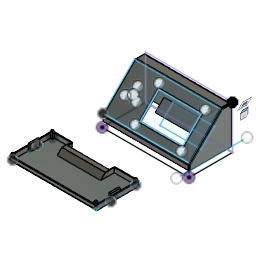
aether pad case split (Autodesk Fusion 360 design; units mm, degrees)
part number: 2026-05-05-17-50-19-673
Autodesk Fusion 360 part; units mm, degrees
sketch "Sketch1" plane through (0, 0, 0) normal (0, 0, 1) x (1, 0, 0)
  line L0 (0, 0) -> (180, 0)
  line L1 (180, 0) -> (180, 90)
  line L2 (180, 90) -> (0, 90)
  line L3 (0, 90) -> (0, 0)
  dimension "d1" = 180
  dimension "d2" = 90
  constraint horizontal L0
  constraint vertical L1
  constraint horizontal L2
  constraint vertical L3
  constraint coincident L0.start L3.end
  measures "d1" distance of L0.start L0.end
  measures "d2" distance of L0.start L2.end
extrude "Extrude1" add sketch "Sketch1" along normal blind 90 makes body 1
sketch "Sketch2" plane through (180, 0, 0) normal (1, 0, 0) x (0, 1, 0)
  line L0 (0, 0) -> (90, 0)
  line L1 (90, 0) -> (90, 90)
  line L2 (90, 90) -> (0, 90)
  line L3 (0, 90) -> (0, 0)
  line L4 (0, 0) -> (0, 22)
  line L5 (90, 90) -> (68, 90)
  line L6 (68, 90) -> (0, 22)
  line L7 (-26.1223, 11.6152) -> (120, 11.6152)
  dimension "d5" = 22
  dimension "d6" = 22
  dimension "d7" = 96.1665
  constraint coincident L0.start L3.end
  constraint perpendicular L0 L4
  constraint coincident L1.end L2.start
  constraint perpendicular L1 L5
  constraint perpendicular L1 L7
  measures "d5" distance of L0.start L4.end
  measures "d6" distance of L1.end L5.end
  measures "d7" distance of L4.end L5.end
extrude "Extrude2" cut sketch "Sketch2" against normal blind 180 contours L2 L3 L6 bodies 1
shell "Shell2" thickness 2 removed faces 0 bodies 1
fillet "Fillet1" radius 2 2 edges at (90, 0, 22) (90, 68, 90) on bodies 1
sketch "Sketch3" plane through (0, -11, 11) normal (0, -0.707107, 0.707107) x (1, 0, 0)
  line L0 (180, 110.8944) -> (0, 110.8944)
  line L1 (0, 110.8944) -> (0, 16.3848)
  line L2 (0, 16.3848) -> (180, 16.3848)
  line L3 (180, 16.3848) -> (180, 110.8944)
  line L4 (0, 18.2322) -> (180, 18.2322)
  line L5 (180, 110.2322) -> (0, 110.2322)
  line L6 (180, 18.2322) -> (180, 110.2322)
  circle A0 centre (17.8756, 57.2322) radius 1.5
  circle A1 centre (42.1244, 57.2322) radius 1.5
  circle A2 centre (60.5, 27.7322) radius 3
  circle A3 centre (30, 64.2322) radius 10
  line L7 (0, 110.2322) -> (0, 18.2322)
  circle A4 centre (30, 78.2322) radius 1.5
  line L8 (65, 89.4322) -> (153, 89.4322)
  circle A5 centre (156, 27.7322) radius 3
  line L9 (65, 35.4322) -> (65, 89.4322)
  circle A6 centre (60.5, 97.7322) radius 3
  line L10 (153, 89.4322) -> (153, 35.4322)
  line L11 (153, 35.4322) -> (65, 35.4322)
  circle A7 centre (156, 97.7322) radius 3
  point P0 (0, 18.2322)
  dimension "d16" = 360
  dimension "d17" = 180
  dimension "d18" = 92
  dimension "d19" = 88
  dimension "d20" = 54
  dimension "d21" = 65
  dimension "d22" = 17.2
  dimension "d23" = 20
  dimension "d24" = 30
  dimension "d25" = 46
  dimension "d26" = 6
  dimension "d27" = 6
  dimension "d28" = 6
  dimension "d29" = 6
  dimension "d30" = 60.5
  dimension "d31" = 79.5
  dimension "d32" = 156
  dimension "d33" = 79.5
  dimension "d34" = 60.5
  dimension "d35" = 9.5
  dimension "d36" = 9.5
  dimension "d37" = 156
  dimension "d38" = 3
  dimension "d39" = 153
  constraint horizontal L4
  constraint vertical L6
  constraint horizontal L5
  constraint vertical L7
  constraint coincident P0 L4.start
  constraint horizontal L8
  constraint vertical L10
  constraint horizontal L11
  constraint vertical L9
  measures "d17" distance of P0 L4.end
  measures "d18" distance of P0 L5.end
  measures "d19" distance of L8.end L8.start
  measures "d20" distance of L8.start L9.start
  measures "d21" distance of L7 L9
  measures "d22" distance of L4 L11
  measures "d23" diameter of A3
  measures "d24" distance of A3.centre L7
  measures "d25" distance of A3.centre L4
  measures "d26" diameter of A6
  measures "d27" diameter of A7
  measures "d28" diameter of A2
  measures "d29" diameter of A5
  measures "d30" distance of A6.centre L7
  measures "d31" distance of A6.centre L4
  measures "d32" distance of A7.centre L7
  measures "d33" distance of A7.centre L4
  measures "d34" distance of A2.centre L7
  measures "d35" distance of A2.centre L4
  measures "d36" distance of A5.centre L4
  measures "d37" distance of A5.centre L7
  measures "d38" diameter of A4
  measures "d39" distance of L7 L10
extrude "Extrude3" cut sketch "Sketch3" against normal blind 3 contours L8 L9 L10 L11 bodies 1
extrude "Extrude4" cut sketch "Sketch3" against normal blind 2 contours A3 bodies 1
extrude "Extrude5" cut sketch "Sketch3" against normal blind 2 contours A0 | A1 | A4 bodies 1
extrude "Extrude6" add sketch "Sketch3" against normal blind 7 contours A2 | A5 | A6 | A7 bodies 1
sketch "Sketch4" plane through (0, 90, 0) normal (0, 1, 0) x (-1, 0, 0)
  line L0 (0, 90) -> (-180, 90)
  line L1 (-180, 0) -> (0, 0)
  line L2 (-180, 90) -> (-180, 0)
  line L3 (0, 0) -> (0, 90)
sketch "Sketch5" plane through (0, 90, 0) normal (0, 1, 0) x (-1, 0, 0)
  line L0 (-130, 0) -> (-40, 0)
  line L1 (-40, 0) -> (-40, 30)
  line L2 (-40, 30) -> (-130, 30)
  line L3 (-130, 30) -> (-130, 0)
  constraint horizontal L0
  constraint vertical L1
  constraint horizontal L2
  constraint vertical L3
extrude "Extrude7" add sketch "Sketch5" against normal blind 30 bodies 1
sketch "Sketch6" plane through (130, 0, 0) normal (1, 0, 0) x (0, 1, 0)
  line L0 (88, 30) -> (60, 30)
  line L1 (60, 30) -> (60, 2)
  line L2 (87.5, 30) -> (88, 30)
  line L3 (88, 30) -> (60, 2)
  line L4 (60, 2) -> (88, 2)
  line L5 (88, 2) -> (88, 30)
  constraint coincident L0 L2.start
  constraint coincident L0.start L2.end
  constraint coincident L1.end L3.end
extrude "Extrude8" cut sketch "Sketch6" against normal blind 90 contours L0 L1 L2 L3 bodies 1
ref_plane "WorkPlane1" through (90, 90, 0) normal (0, -0.707107, 0.707107) x (-1, 0, 0)
sketch "Sketch7" plane through (0, 45, -45) normal (0, -0.707107, 0.707107) x (-1, 0, 0)
  line L0 (-128.5484, -83.2783) -> (-42.857, -83.2783)
  line L1 (-42.857, -83.2783) -> (-42.857, -44.6734)
  line L2 (-42.857, -44.6734) -> (-128.5484, -44.6734)
  line L3 (-128.5484, -44.6734) -> (-128.5484, -83.2783)
  constraint horizontal L0
  constraint vertical L1
  constraint horizontal L2
  constraint vertical L3
extrude "Extrude11" cut sketch "Sketch7" along normal blind 16 bodies 1
fillet "Fillet5" radius 5 1 edges at (90, 0, 0) on bodies 1
fillet "Fillet6" radius 5 3 edges at (21.4285, 90, 0) (154.2742, 90, 0) (90, 90, 90) on bodies 1
fillet "Fillet7" radius 2 8 edges at (85.7027, 67.3726, 0) (128.5484, 76.1863, 0) (128.5484, 88.5355, 1.4645) (128.5484, 90, 13.8137) (85.7027, 90, 22.6274) (42.857, 90, 13.8137) (42.857, 88.5355, 1.4645) (42.857, 76.1863, 0) on bodies 1
fillet "Fillet8" radius 2 10 edges at (180, 90, 45) (180, 88.5355, 1.4645) (180, 45, 0) (180, 1.4645, 1.4645) (180, 0, 13.0858) (180, 0.1522, 21.9369) (180, 34, 56) (180, 68.0631, 89.8478) (180, 76.9142, 90) (180, 88.5355, 88.5355) on bodies 1
fillet "Fillet9" radius 2 10 edges at (0, 76.9142, 90) (0, 68.0631, 89.8478) (0, 34, 56) (0, 0.1522, 21.9369) (0, 0, 13.0858) (0, 1.4645, 1.4645) (0, 45, 0) (0, 88.5355, 1.4645) (0, 90, 45) (0, 88.5355, 88.5355) on bodies 1
fillet "Fillet10" radius 2 4 edges at (109, 52.2381, 74.2381) (65, 33.1462, 55.1462) (109, 14.0543, 36.0543) (153, 33.1462, 55.1462) on bodies 1
split "Split1" by curves path "Sketch2" along L7 bodies 1 makes body 2 at (103.3333, 21.3333, 2)
move_body "Move1" bodies 2 to x (1, 0, 0) y (0, 1, 0) z (0, 0, 1) at (-64.9771, -127.9418, -30.8642)
sketch "Sketch8" plane through (0, 0, -28.8642) normal (0, 0, 1) x (-1, 0, 0)
  line L0 (-65.0229, 39.9418) -> (-65.0229, 67.9418)
  line L1 (-65.0229, 67.9418) -> (24.9771, 67.9418)
  line L2 (24.9771, 67.9418) -> (24.9771, 39.9418)
  line L3 (24.9771, 39.9418) -> (62.9771, 39.9418)
  line L4 (62.9771, 39.9418) -> (62.9771, 125.9418)
  line L5 (62.9771, 125.9418) -> (-113.0229, 125.9418)
  line L6 (-113.0229, 125.9418) -> (-113.0229, 39.9418)
  line L7 (-113.0229, 39.9418) -> (-65.0229, 39.9418)
  line L8 (62.9771, 121.9229) -> (58.9771, 121.9229)
  line L9 (58.9771, 121.9229) -> (58.9771, 125.9229)
  line L10 (58.9771, 125.9229) -> (62.9771, 125.9229)
  line L11 (62.9771, 125.9229) -> (62.9771, 121.9229)
  line L12 (-113.0106, 121.9232) -> (-109.0106, 121.9232)
  line L13 (-109.0106, 121.9232) -> (-109.0106, 125.9232)
  line L14 (-109.0106, 125.9232) -> (-113.0106, 125.9232)
  line L15 (-113.0106, 125.9232) -> (-113.0106, 121.9232)
  line L16 (-109.2501, 39.9418) -> (-113.2501, 39.9418)
  line L17 (-113.2501, 39.9418) -> (-113.2501, 43.9418)
  line L18 (-113.2501, 43.9418) -> (-109.2501, 43.9418)
  line L19 (-109.2501, 43.9418) -> (-109.2501, 39.9418)
  line L20 (62.9771, 39.9418) -> (58.9771, 39.9418)
  line L21 (58.9771, 39.9418) -> (58.9771, 43.9418)
  line L22 (58.9771, 43.9418) -> (62.9771, 43.9418)
  line L23 (62.9771, 43.9418) -> (62.9771, 39.9418)
  line L24 (-113.0229, 95.0265) -> (-109.0229, 95.0265)
  line L25 (-109.0229, 95.0265) -> (-109.0229, 75.0265)
  line L26 (-109.0229, 75.0265) -> (-113.0229, 75.0265)
  line L27 (-113.0229, 75.0265) -> (-113.0229, 95.0265)
  line L28 (62.9771, 70.1255) -> (58.9771, 70.1255)
  line L29 (58.9771, 70.1255) -> (58.9771, 90.1255)
  line L30 (58.9771, 90.1255) -> (62.9771, 90.1255)
  line L31 (62.9771, 90.1255) -> (62.9771, 70.1255)
  dimension "d88" = 4
  dimension "d89" = 4
  dimension "d92" = 4
  dimension "d93" = 4
  dimension "d94" = 4
  dimension "d95" = 4
  dimension "d96" = 4
  dimension "d97" = 4
  dimension "d104" = 4
  dimension "d105" = 20
  dimension "d106" = 4
  dimension "d107" = 20
  constraint horizontal L8
  constraint vertical L9
  constraint horizontal L10
  constraint vertical L11
  constraint coincident L4 L8.start
  constraint horizontal L12
  constraint vertical L13
  constraint horizontal L14
  constraint vertical L15
  constraint horizontal L16
  constraint vertical L17
  constraint horizontal L18
  constraint vertical L19
  constraint coincident L7 L16.start
  constraint horizontal L20
  constraint vertical L21
  constraint horizontal L22
  constraint vertical L23
  constraint coincident L3.end L4.start
  constraint horizontal L24
  constraint vertical L25
  constraint horizontal L26
  constraint vertical L27
  constraint coincident L6 L24.start
  constraint horizontal L28
  constraint vertical L29
  constraint horizontal L30
  constraint vertical L31
  constraint coincident L4 L28.start
  measures "d88" distance of L8.start L8.end
  measures "d89" distance of L8.start L10.end
  measures "d92" distance of L12.start L12.end
  measures "d93" distance of L12.start L14.end
  measures "d94" distance of L16.start L16.end
  measures "d95" distance of L16.start L18.end
  measures "d96" distance of L3.end L20.end
  measures "d97" distance of L3.end L22.end
  measures "d104" distance of L24.start L24.end
  measures "d105" distance of L24.start L26.end
  measures "d106" distance of L28.start L28.end
  measures "d107" distance of L28.start L30.end
extrude "Extrude12" add sketch "Sketch8" along normal blind 14 contours L4 L8 L9 L10 L11 bodies 2
extrude "Extrude13" add sketch "Sketch8" along normal blind 14 contours L3 L4 L20 L21 L22 L23 bodies 2
sketch "Sketch9" plane through (115.0229, 0, 0) normal (1, 0, 0) x (0, 1, 0)
  line L0 (-39.9418, -19.249) -> (-125.9418, -19.249)
  line L1 (-125.9418, -19.249) -> (-125.9418, -25.8642)
  arc A0 (-125.9418, -25.8642) -> (-122.9418, -28.8642) centre (-122.9418, -25.8642) ccw
  line L2 (-122.9418, -28.8642) -> (-42.9418, -28.8642)
  arc A1 (-42.9418, -28.8642) -> (-39.9418, -25.8642) centre (-42.9418, -25.8642) ccw
  line L3 (-39.9418, -25.8642) -> (-39.9418, -19.249)
extrude "Extrude14" add sketch "Sketch8" along normal blind 14 contours L6 L7 L16 L18 L19 bodies 2
extrude "Extrude15" add sketch "Sketch8" along normal blind 14 contours L12 L13 L14 L15 bodies 2
extrude "Extrude16" add sketch "Sketch8" along normal blind 14 contours L4 L28 L29 L30 L31 bodies 2
extrude "Extrude17" add sketch "Sketch8" along normal blind 14 contours L6 L24 L25 L26 L27 bodies 2
equation "d5 = d6"
equation "d30 = d34"
equation "d31 = d33"
equation "d35 = d36"
